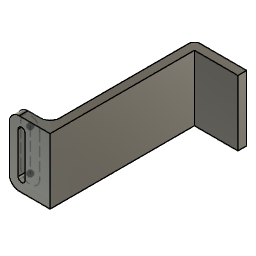
battery_clip v1 (Autodesk Fusion 360 design; units mm, degrees)
Autodesk Fusion 360 part; units mm, degrees
sketch "Sketch1" plane through (0, 0, 0) normal (0, 0, 1) x (1, 0, 0)
  line L0 (0, 0) -> (0, 4)
  line L1 (0, 4) -> (14.7, 4)
  line L2 (14.7, 4) -> (14.7, 70.3)
  line L3 (14.7, 70.3) -> (38.7, 70.3)
  line L4 (38.7, 70.3) -> (38.7, 66.3)
  line L5 (38.7, 66.3) -> (18.7, 66.3)
  line L6 (18.7, 66.3) -> (18.7, 0)
  line L7 (18.7, 0) -> (0, 0)
  dimension "d7" = 4
  dimension "d8" = 4
  dimension "d9" = 4
  dimension "d10" = 66.3
  dimension "d11" = 20
  dimension "d12" = 14.7
  constraint coincident L0.start L7.end
  constraint vertical L0
  constraint perpendicular L0 L1
  constraint perpendicular L1 L2
  constraint perpendicular L2 L3
  constraint perpendicular L3 L4
  constraint perpendicular L4 L5
  constraint perpendicular L5 L6
  constraint perpendicular L0 L7
  measures "d7" distance of L1 L7
  measures "d8" distance of L2 L6
  measures "d9" distance of L3 L5
  measures "d10" distance of L5 L7
  measures "d11" distance of L4.end L5.end
  measures "d12" distance of L0.end L1.end
extrude "Extrude1" add sketch "Sketch1" along normal blind 30
sketch "Sketch2" plane through (0, 4, 0) normal (0, 1, 0) x (-1, 0, 0)
  line L0 (-14.7, 0) -> (0, 0)
  line L1 (0, 0) -> (0, 30)
  line L2 (0, 30) -> (-14.7, 30)
  line L3 (-14.7, 30) -> (-14.7, 0)
  line L4 (-7.2, 24.4) -> (-7.2, 5.6)
  arc A0 (-7.2, 5.6) -> (-4, 5.6) centre (-5.6, 5.6) ccw
  line L5 (-4, 5.6) -> (-4, 24.4)
  arc A1 (-4, 24.4) -> (-7.2, 24.4) centre (-5.6, 24.4) ccw
  line L6 (-5.6, 24.4) -> (-5.6, 5.6) construction
  line L7 (-5.6, 24.4) -> (-5.6, 30) construction
  line L8 (-5.6, 5.6) -> (-5.6, 0) construction
  point P0 (-5.6, 26)
  dimension "d16" = 1.6
  dimension "d17" = 4
  dimension "d18" = 4
  constraint tangent L4 A0
  constraint tangent A0 L5
  constraint parallel L4 L5
  constraint tangent L5 A1
  constraint tangent L4 A1
  constraint parallel L3 L6
  constraint coincident A1.centre L6.start
  constraint coincident L2 L7.end
  constraint coincident A0.centre L6.end
  constraint coincident L0 L8.end
  constraint vertical L7
  constraint vertical L8
  constraint equal L7 L8
  constraint midpoint A1 P0
  measures "d16" radius of A1
  measures "d17" distance of L1 L5
  measures "d18" distance of L2 P0
extrude "Extrude2" cut sketch "Sketch2" against normal up to surface (4 mm away) contours L4 A0 L5 A1
fillet "Fillet1" radius 2.5 1 edges at (14.7, 70.3, 15)
fillet "Fillet2" radius 4.5 2 edges at (0, 2, 30) (0, 2, 0)
sketch "Sketch3" plane through (0, 4, 0) normal (0, 1, 0) x (-1, 0, 0)
  arc A0 (-4.5, 0) -> (0, 4.5) centre (-4.5, 4.5) ccw
  line L0 (0, 4.5) -> (0, 25.5)
  arc A1 (0, 25.5) -> (-4.5, 30) centre (-4.5, 25.5) ccw
  line L1 (-4.5, 30) -> (-14.7, 30)
  line L2 (-14.7, 30) -> (-14.7, 0)
  line L3 (-14.7, 0) -> (-4.5, 0)
  arc A2 (-4, 24.4) -> (-7.2, 24.4) centre (-5.6, 24.4) ccw
  line L4 (-4, 24.4) -> (-4, 5.6)
  arc A3 (-7.2, 5.6) -> (-4, 5.6) centre (-5.6, 5.6) ccw
  line L5 (-7.2, 5.6) -> (-7.2, 24.4)
  line L6 (-9.95, 24.4) -> (-9.95, 5.6) construction
  arc A4 (-9.95, 5.6) -> (-1.25, 5.6) centre (-5.6, 5.6) ccw construction
  line L7 (-1.25, 5.6) -> (-1.25, 24.4) construction
  arc A5 (-1.25, 24.4) -> (-9.95, 24.4) centre (-5.6, 24.4) ccw construction
  line L8 (-5.6, 24.4) -> (-5.6, 5.6) construction
  dimension "d25" = 4.35
  constraint tangent L6 A4
  constraint tangent A4 L7
  constraint parallel L6 L7
  constraint tangent L7 A5
  constraint tangent L6 A5
  constraint coincident A3.centre A4.centre
  constraint parallel L4 L8
  constraint coincident A2.centre A5.centre
  measures "d25" radius of A5
fillet "Fillet3" radius 4.5 1 edges at (14.7, 4, 15)
equation "batt_depth = 65.5 mm"
equation "M3_D = 3 mm"
equation "clearance = 0.2 mm"
equation "clip_W = 30 mm"
equation "clip_overhang = 20 mm"
equation "clip_t = 4 mm"
equation "d7 = clip_t"
equation "d8 = d7"
equation "d9 = d7"
equation "d10 = batt_depth + clearance * 4"
equation "d11 = clip_overhang"
equation "d12 = M4_washer_D + 2 mm + clip_t"
equation "M4_washer_D = 8.7 mm"
equation "d14 = clip_W"
equation "d16 = ( M3_D + clearance ) / 2"
equation "d17 = clip_t"
equation "d18 = clip_t"
equation "d25 = M4_washer_D / 2"
